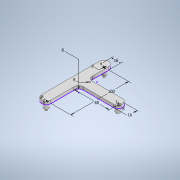
# Autodesk Inventor part: Practica 8
Saved by Autodesk Inventor 2020 (Build 240168000, 168)
## iProperties
Created: 2020-02-22
Part Number: Practica 8
Material: Genérico
Document SubType Name: Modeling
Designer: luisg
Density: 1 g/cm^3
Appearance: Valor por defecto
Author: luisg
Autodesk Inventor part; units mm, degrees
ref_plane "YZ Plane" through (0, 0, 0) normal (1, 0, 0) x (0, 1, 0)
ref_plane "XZ Plane" through (0, 0, 0) normal (0, 1, 0) x (-1, 0, 0)
ref_plane "XY Plane" through (0, 0, 0) normal (0, 0, 1) x (1, 0, 0)
sketch "Boceto1" plane through (0, 0, 0) normal (0, 1, 0) x (-1, 0, 0)
  line L0 (0, -100) -> (0, 0)
  line L1 (-76, -48) -> (-24, -48)
  line L2 (-24, -64) -> (-76, -64)
  arc A0 (-16, -100) -> (0, -100) centre (-8, -100) ccw
  arc A1 (0, 0) -> (-16, 0) centre (-8, 0) ccw
  arc A2 (-76, -48) -> (-76, -64) centre (-76, -56) ccw
  line L3 (-16, 0) -> (-16, -40)
  line L4 (-16, -72) -> (-16, -100)
  arc A3 (-24, -48) -> (-16, -40) centre (-24, -40) ccw
  arc A4 (-16, -72) -> (-24, -64) centre (-24, -72) ccw
  circle A5 centre (-8, 0) radius 4
  circle A6 centre (-8, -100) radius 4
  circle A7 centre (-76, -56) radius 4
  circle A8 centre (-76, -58) radius 0.5
  circle A9 centre (-76, -54) radius 0.5
  circle A10 centre (-8, -100) radius 2
  circle A11 centre (-8, 0) radius 2
  point P0 (-16, -48)
  dimension "d0" = 16
  dimension "d1" = 100
  dimension "d2" = 60
  dimension "d3" = 16
  dimension "d6" = 8
  dimension "d7" = 8
  dimension "d8" = 8
  dimension "d9" = 8
  dimension "d10" = 8
  dimension "d11" = 8
  dimension "d12" = 8
  dimension "d13" = 1
  dimension "d14" = 1
  dimension "d15" = 2
  dimension "d16" = 2
  dimension "d17" = 4
  dimension "d18" = 4
  constraints: 12 centre point, 10 end point, 10 point on circle, 5 coincident, 4 tangent, 3 parallel, 2 point on line, 1 horizontal
  measures "d0" distance of L0.start L4.end
  measures "d1" distance of L3.start L4.end
  measures "d2" distance of point (-16, -48) L1.start
  measures "d3" distance of L2.end L1.start
  measures "d6" radius of A1
  measures "d7" radius of A2
  measures "d8" radius of A3
  measures "d9" radius of A4
  measures "d10" diameter of A5
  measures "d11" diameter of A6
  measures "d12" diameter of A7
  measures "d13" diameter of A8
  measures "d14" diameter of A9
  measures "d15" distance of A8.centre A2.centre
  measures "d16" distance of A2.centre A9.centre
  measures "d17" diameter of A10
  measures "d18" diameter of A11
extrude "Extrusión1" add sketch "Boceto1" along normal blind 5 contours A0 L4 A4 L2 A2 L1 A3 L3 A1 L0 | A5 | A6 | A7 | A8 | A9 | A10 | A11
sketch "Boceto4" plane through (0, 0, 0) normal (0, -1, 0) x (1, 0, 0)
  point P0 (0, 0)
extrude "Extrusión3" add sketch "Boceto1" against normal blind 14 contours A10 | A11
sketch "Boceto5" plane through (0, 0, 0) normal (0, -1, 0) x (1, 0, 0)
  point P0 (0, 0)
extrude "Extrusión4" add sketch "Boceto1" against normal blind 12 contours A8 | A9
sketch "Boceto6" plane through (0, 0, 0) normal (0, -1, 0) x (1, 0, 0)
  point P0 (0, 0)
extrude "Extrusión5" add sketch "Boceto1" against normal blind 10 contours A5 | A6 | A7 | A10 | A11
